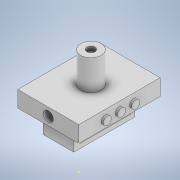
# Autodesk Inventor part: body (2)
Saved by Autodesk Inventor 2021 (Build 250183000, 183)
## iProperties
Created: 2021-07-08
Part Number: body (2)
Material: Generic
Document SubType Name: Modeling
Designer: 91968
Density: 1 g/cm^3
Appearance: Default
Author: 91968
Autodesk Inventor part; units mm, degrees
ref_plane "YZ Plane" through (0, 0, 0) normal (1, 0, 0) x (0, 1, 0)
ref_plane "XZ Plane" through (0, 0, 0) normal (0, 1, 0) x (-1, 0, 0)
ref_plane "XY Plane" through (0, 0, 0) normal (0, 0, 1) x (1, 0, 0)
sketch "Sketch1" plane through (0, 0, 0) normal (1, 0, 0) x (0, 1, 0)
  line L0 (0, 0) -> (80, 0)
  line L1 (80, 0) -> (80, -400)
  line L2 (80, -400) -> (0, -400)
  line L3 (0, -400) -> (0, 0)
  dimension "d0" = 80
  dimension "d1" = 400
  constraints: 8 end point, 2 parallel, 1 horizontal, 1 perpendicular
  measures "d0" distance of L1.end L2.end
  measures "d1" distance of L0.end L1.end
extrude "Extrusion1" add sketch "Sketch1" against normal blind 300
sketch "Sketch2" plane through (0, 0, 0) normal (1, 0, 0) x (0, 0, -1)
  circle A0 centre (130, 36.5604) radius 20
  circle A1 centre (200, 36.5604) radius 20
  circle A2 centre (270, 36.5604) radius 20
  line L0 (0, 80) -> (0, 0) projected
  line L1 (400, 0) -> (400, 80) projected
  dimension "d4" = 40
  dimension "d5" = 40
  dimension "d6" = 40
  dimension "d7" = 130
  dimension "d8" = 130
  dimension "d9" = 70
  constraints: 3 centre point
  measures "d4" diameter of A0
  measures "d5" diameter of A1
  measures "d6" diameter of A2
  measures "d7" distance from line of A0.centre L0
  measures "d8" distance from line of L1 A2.centre
  measures "d9" distance of A1.centre A0.centre
extrude "Extrusion2" add sketch "Sketch2" along normal blind 10 contours A0
extrude "Extrusion3" add sketch "Sketch2" along normal blind 10 contours A1
extrude "Extrusion4" add sketch "Sketch2" along normal blind 10 contours A2
sketch "Sketch3" plane through (0, 80, 0) normal (0, 1, 0) x (1, 0, 0)
  circle A0 centre (-140.3312, 200) radius 50
  line L0 (0, 0) -> (-300, 0) projected
  dimension "d16" = 100
  dimension "d17" = 200
  constraints: 1 centre point
  measures "d16" diameter of A0
  measures "d17" distance from line of A0.centre L0
extrude "Extrusion5" add sketch "Sketch3" along normal blind 150
sketch "Sketch4" plane through (-140.3312, 230, -200) normal (0, 1, 0) x (1, 0, 0)
  circle A0 centre (0, 0) radius 20
  point P0 (140.3312, -200)
  dimension "d20" = 40
  constraints: 1 centre point
  measures "d20" diameter of A0
extrude "Extrusion6" cut sketch "Sketch4" against normal blind 20
sketch "Sketch5" plane through (0, 0, -400) normal (0, -1, 0) x (1, 0, 0)
  line L0 (-75, 350) -> (-75, 50)
  line L1 (-75, 50) -> (-225, 50)
  line L2 (-225, 50) -> (-225, 350)
  line L3 (-225, 350) -> (-75, 350)
  line L4 (0, 400) -> (0, 0) projected
  line L5 (0, 0) -> (-300, 0) projected
  dimension "d23" = 300
  dimension "d24" = 150
  dimension "d25" = 300
  dimension "d26" = 75
  dimension "d27" = 50
  constraints: 8 end point, 2 perpendicular, 1 vertical
  measures "d23" distance of L0.start L0.end
  measures "d24" distance of L0.end L1.end
  measures "d25" distance of L1.end L2.end
  measures "d26" distance between parallel lines of L0 L4
  measures "d27" distance between parallel lines of L5 L1
sketch "Sketch6" plane through (0, 0, -400) normal (0, -1, 0) x (1, 0, 0)
  point P0 (0, 400)
extrude "Extrusion7" add sketch "Sketch5" along normal blind 100
sketch "Sketch7" plane through (0, -100, -400) normal (0, -1, 0) x (1, 0, 0)
  circle A0 centre (-150, 200) radius 30
  line L0 (-225, 50) -> (-75, 50) projected
  line L1 (-75, 50) -> (-75, 350) projected
  point P0 (0, 400)
  dimension "d30" = 60
  dimension "d31" = 150
  dimension "d32" = 75
  constraints: 1 centre point
  measures "d30" diameter of A0
  measures "d31" distance from line of A0.centre L0
  measures "d32" distance from line of A0.centre L1
extrude "Extrusion8" add sketch "Sketch7" along normal blind 20
sketch "Sketch8" plane through (-150, -120, -200) normal (0, -1, 0) x (1, 0, 0)
  point P0 (150, 200)
sketch "Sketch9" plane through (0, 0, 0) normal (0, 0, 1) x (1, 0, 0)
  circle A0 centre (-150, 40) radius 25
  line L0 (-300, 0) -> (-300, 80) projected
  line L1 (0, 80) -> (-300, 80) projected
  point P0 (0, 0)
  dimension "d35" = 50
  dimension "d36" = 150
  dimension "d37" = 40
  constraints: 1 centre point
  measures "d35" diameter of A0
  measures "d36" distance from line of A0.centre L0
  measures "d37" distance from line of A0.centre L1
extrude "Extrusion9" cut sketch "Sketch9" against normal blind 50
sketch "Sketch10" plane through (0, 0, -400) normal (0, 0, -1) x (-1, 0, 0)
  circle A0 centre (150, 40) radius 25 projected
  circle A1 centre (150, 40) radius 25
  point P0 (0, 0)
  constraints: 1 centre point, 1 coincident
extrude "Extrusion10" cut sketch "Sketch10" against normal blind 50
sketch "Sketch11" plane through (-75, 0, -50) normal (1, 0, 0) x (0, 0, -1)
  line L0 (29.0215, -18.1816) -> (279.0215, -18.1816)
  line L1 (279.0215, -18.1816) -> (279.0215, -78.1816)
  line L2 (279.0215, -78.1816) -> (29.0215, -78.1816)
  line L3 (29.0215, -78.1816) -> (29.0215, -18.1816)
  point P0 (-50, 0)
  dimension "d42" = 250
  dimension "d43" = 60
  constraints: 8 end point, 2 parallel, 1 horizontal, 1 perpendicular
  measures "d42" distance of L1.end L2.end
  measures "d43" distance of L0.end L1.end
extrude "Extrusion11" cut sketch "Sketch11" against normal blind 10
fillet "Fillet1" radius 4 4 edges at (-85, -48.1816, -329.0215) (-85, -18.1816, -204.0215) (-85, -78.1816, -204.0215) (-85, -48.1816, -79.0215)
sketch "Sketch12" plane through (-300, 0, 0) normal (-1, 0, 0) x (0, 0, 1)
  line L0 (-20.388, 18.3372) -> (-370.388, 18.3372)
  line L1 (-370.388, 18.3372) -> (-370.388, 58.3372)
  line L2 (-370.388, 58.3372) -> (-20.388, 58.3372)
  line L3 (-20.388, 58.3372) -> (-20.388, 18.3372)
  point P0 (0, 0)
  dimension "d47" = 350
  dimension "d48" = 40
  constraints: 8 end point, 2 parallel, 1 horizontal, 1 perpendicular
  measures "d47" distance of L1.end L2.end
  measures "d48" distance of L0.end L1.end
extrude "Extrusion12" cut sketch "Sketch12" against normal blind 10
fillet "Fillet2" radius 2 4 edges at (-290, 18.3372, -195.388) (-290, 38.3372, -370.388) (-290, 38.3372, -20.388) (-290, 58.3372, -195.388)
sketch "Sketch13" plane through (-85, 0, -50) normal (1, 0, 0) x (0, 0, -1)
  circle A0 centre (146.4262, -46.2866) radius 20
  point P0 (-50, 0)
  dimension "d52" = 40
  constraints: 1 centre point
  measures "d52" diameter of A0
extrude "Extrusion13" cut sketch "Sketch13" against normal blind 100
body "Solid1"
